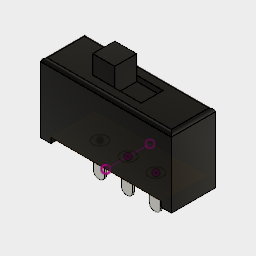
805 SPDT Breadboard Friendly Slide Switch (Autodesk Fusion 360 design; units mm, degrees)
Autodesk Fusion 360 part; units mm, degrees
sketch "Slider" plane through (0, 0, 0) normal (0, 0, 1) x (1, 0, 0)
  line L0 (0, 0) -> (11.9, 0)
  line L1 (11.9, 0) -> (11.9, -4)
  line L2 (11.9, -4) -> (0, -4)
  line L3 (0, -4) -> (0, 0)
  line L4 (5.95, 0) -> (5.95, -4) construction
  line L5 (0, -2) -> (11.9, -2) construction
  line L6 (8.15, -3) -> (3.75, -3)
  line L7 (3.75, -3) -> (3.75, -1)
  line L8 (3.75, -1) -> (8.15, -1)
  line L9 (8.15, -1) -> (8.15, -3)
  line L10 (8.15, -3) -> (3.75, -1) construction
  line L11 (3.75, -3) -> (8.15, -1) construction
  line L12 (3.75, -1) -> (5.75, -1)
  line L13 (5.75, -1) -> (5.75, -3)
  line L14 (5.75, -3) -> (3.75, -3)
  line L15 (3.75, -3) -> (3.75, -1)
  point P0 (5.95, -2)
  dimension "d1" = 11.9
  dimension "d2" = 4
  dimension "d3" = 4.4
  dimension "d4" = 2
  dimension "d5" = 2
  measures "d1" distance of L0.start L0.end
  measures "d2" distance of L0.start L2.end
  measures "d3" distance of L7.end L8.end
  measures "d4" distance of L6.end L7.end
  measures "d5" distance of L7.end L12.end
extrude "Extrude1" add sketch "Slider" against normal blind 6.3 contours L0 L1 L2 L3 | L6 L8 L9 L13 | L6 L7 L8 L12 L13 L14 L15 makes body 1
extrude "Extrude2" cut sketch "Slider" against normal blind 0.5 contours L6 L8 L9 L13 | L6 L7 L8 L12 L13 L14 L15 bodies 1
extrude "Extrude3" add sketch "Slider" along normal blind 1.7 and the other way blind 0.5 contours L6 L7 L8 L12 L13 L14 L15 bodies 1
sketch "Base" plane through (0, 0, -6.3) normal (0, 0, -1) x (1, 0, 0)
  line L0 (11.9, 4) -> (0, 4)
  line L1 (0, 4) -> (0, 0)
  line L2 (0, 0) -> (11.9, 0)
  line L3 (11.9, 0) -> (11.9, 4)
  line L4 (5.95, 4) -> (5.95, 0) construction
  line L5 (0, 2) -> (11.9, 2) construction
  line L6 (10.95, 0) -> (0.95, 0)
  line L7 (0.95, 0) -> (0.95, 4)
  line L8 (0.95, 4) -> (10.95, 4)
  line L9 (10.95, 4) -> (10.95, 0)
  line L10 (10.95, 0) -> (0.95, 4) construction
  line L11 (0.95, 0) -> (10.95, 4) construction
  point P0 (5.95, 2)
  dimension "d13" = 10
  dimension "d14" = 4
  measures "d13" distance of L7.end L8.end
  measures "d14" distance of L6.end L7.end
extrude "Extrude4" cut sketch "Base" against normal blind 0.5 contours L0 L2 L6 L7 L8 L9 bodies 1
sketch "Pins" plane through (0, 0, -5.8) normal (0, 0, -1) x (1, 0, 0)
  line L0 (10.95, 4) -> (0.95, 4)
  line L1 (0.95, 4) -> (0.95, 0)
  line L2 (0.95, 0) -> (10.95, 0)
  line L3 (10.95, 0) -> (10.95, 4)
  line L4 (5.95, 4) -> (5.95, 0) construction
  line L5 (10.95, 2) -> (0.95, 2) construction
  line L6 (6.45, 2.1) -> (5.45, 2.1)
  line L7 (5.45, 2.1) -> (5.45, 1.9)
  line L8 (5.45, 1.9) -> (6.45, 1.9)
  line L9 (6.45, 1.9) -> (6.45, 2.1)
  line L10 (6.45, 2.1) -> (5.45, 1.9) construction
  line L11 (5.45, 2.1) -> (6.45, 1.9) construction
  line L12 (8.99, 2.1) -> (7.99, 2.1)
  line L13 (7.99, 2.1) -> (7.99, 1.9)
  line L14 (7.99, 1.9) -> (8.99, 1.9)
  line L15 (8.99, 1.9) -> (8.99, 2.1)
  line L16 (8.99, 2.1) -> (7.99, 1.9) construction
  line L17 (7.99, 2.1) -> (8.99, 1.9) construction
  line L18 (3.91, 1.9) -> (2.91, 1.9)
  line L19 (2.91, 2.1) -> (3.91, 2.1)
  line L20 (2.91, 1.9) -> (2.91, 2.1)
  line L21 (3.91, 2.1) -> (3.91, 1.9)
  point P0 (5.95, 2)
  point P1 (8.49, 2)
  dimension "d18" = 1
  dimension "d19" = 0.2
  dimension "d20" = 0.2
  dimension "d21" = 1
  dimension "d22" = 2.54
  measures "d18" distance of L7.end L8.end
  measures "d19" distance of L6.end L7.end
  measures "d20" distance of L12.end L13.end
  measures "d21" distance of L13.end L14.end
  measures "d22" distance of P0 P1
extrude "Extrude5" add sketch "Pins" along normal blind 3 separate body contours L6 L7 L8 L9 | L12 L13 L14 L15 | L18 L19 L20 L21 makes body 2 at (3.2433, -1.9, -7.8) makes body 3 at (5.7833, -1.9, -6.8) makes body 4 at (8.3233, -1.9, -6.8)
fillet "Fillet1" radius 0.45 6 edges at (8.99, -2, -8.8) (7.99, -2, -8.8) (6.45, -2, -8.8) (5.45, -2, -8.8) (3.91, -2, -8.8) (2.91, -2, -8.8) on bodies 2 3 4
fillet "Fillet2" radius 0.3 4 edges at (0, -2, 0) (5.95, -4, 0) (5.95, 0, 0) (11.9, -2, 0) on bodies 1
sketch "Connections" plane through (0, 0, -5.8) normal (0, 0, -1) x (1, 0, 0)
  line L0 (10.95, 4) -> (0.95, 4)
  line L1 (0.95, 4) -> (0.95, 0)
  line L2 (0.95, 0) -> (10.95, 0)
  line L3 (10.95, 0) -> (10.95, 4)
  circle A0 centre (5.95, 2) radius 0.635
  line L4 (5.95, 4) -> (5.95, 0)
  circle A1 centre (8.49, 2) radius 0.635
  circle A2 centre (3.41, 2) radius 0.635
  point P0 (8.49, 2)
  point P1 (5.95, 2)
  dimension "d28" = 1.27
  dimension "d29" = 1.27
  measures "d28" diameter of A0
  measures "d29" diameter of A1
equation "d20 = d19"
equation "d21 = d18"
equation "WireDia = 1.27 mm"
equation "d28 = WireDia"
equation "d29 = WireDia"
named bodies: "Pin1", "Pin2 Center", "Pin3"
